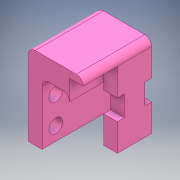
# Autodesk Inventor part: crochet
Saved by Autodesk Inventor 2017 (Build 210142000, 142)
## iProperties
Created: 2017-04-13
Part Number: crochet
Material: Generic
Document SubType Name: Modeling
Designer: franc
Density: 1 g/cm^3
Appearance: Default
Author: franc
Autodesk Inventor part; units mm, degrees
ref_plane "YZ Plane" through (0, 0, 0) normal (1, 0, 0) x (0, 1, 0)
ref_plane "XZ Plane" through (0, 0, 0) normal (0, 1, 0) x (-1, 0, 0)
ref_plane "XY Plane" through (0, 0, 0) normal (0, 0, 1) x (1, 0, 0)
sketch "Sketch1" plane through (0, 0, 0) normal (0, 1, 0) x (-1, 0, 0)
  line L0 (-4.0561, -5.7426) -> (-4.0561, 5.2574)
  line L1 (-3.0561, 6.2574) -> (2.9439, 6.2574)
  line L2 (3.9439, 5.2574) -> (3.9439, -5.7426)
  line L3 (3.9439, -5.7426) -> (1.9439, -5.7426)
  line L4 (1.9439, -5.7426) -> (1.9439, 2.2574)
  line L5 (0.9439, 3.2574) -> (-1.0561, 3.2574)
  line L6 (-2.0561, 2.2574) -> (-2.0561, -5.7426)
  line L7 (-2.0561, -5.7426) -> (-4.0561, -5.7426)
  arc A0 (-1.0561, 3.2574) -> (-2.0561, 2.2574) centre (-1.0561, 2.2574) ccw
  arc A1 (1.9439, 2.2574) -> (0.9439, 3.2574) centre (0.9439, 2.2574) ccw
  arc A2 (-3.0561, 6.2574) -> (-4.0561, 5.2574) centre (-3.0561, 5.2574) ccw
  arc A3 (3.9439, 5.2574) -> (2.9439, 6.2574) centre (2.9439, 5.2574) ccw
  point P0 (0, 0)
  point P1 (-4.0561, 6.2574)
  point P2 (3.9439, 6.2574)
  point P3 (1.9439, 3.2574)
  point P4 (-2.0561, 3.2574)
  dimension "d0" = 12
  dimension "d1" = 2
  dimension "d2" = 2
  dimension "d3" = 8
  dimension "d4" = 3
  dimension "d20" = 1
  constraints: 16 end point, 9 point on line, 8 point on circle, 8 tangent, 7 perpendicular, 4 centre point, 3 equal radius, 1 vertical
  measures "d0" distance of L0.start point (-4.056, 6.257)
  measures "d1" distance of L6.end L0.start
  measures "d2" distance of L2.end L3.end
  measures "d3" distance of point (-4.056, 6.257) point (3.944, 6.257)
  measures "d4" distance between parallel lines of L1 L5
  measures "d20" radius of A0
extrude "Extrusion1" add sketch "Sketch1" along normal blind 10
sketch "Sketch6" plane through (-1.9439, 0, 2.2574) normal (1, 0, 0) x (0, 0, -1)
  circle A0 centre (2, 2) radius 1
  circle A1 centre (6, 2) radius 1
  line L0 (8, 0) -> (8, 10) projected
  line L1 (0, 10) -> (8, 10) projected
  line L2 (8, 0) -> (0, 0) projected
  point P0 (2.2574, 0)
  dimension "d44" = 2
  dimension "d45" = 2
  dimension "d46" = 2
  dimension "d47" = 6
  dimension "d52" = 2
  dimension "d53" = 2
  constraints: 2 centre point
  measures "d44" diameter of A0
  measures "d45" diameter of A1
  measures "d46" distance from line of L0 A1.centre
  measures "d47" distance from line of L0 A0.centre
  measures "d52" distance from line of L2 A0.centre
  measures "d53" distance from line of L2 A1.centre
extrude "Extrusion6" cut sketch "Sketch6" against normal up to next
sketch "Sketch7" plane through (4.0561, 0, 5.2574) normal (1, 0, 0) x (0, 0, -1)
  line L0 (4, 10) -> (4, 9)
  line L1 (4, 9) -> (7, 9)
  line L2 (7, 9) -> (7, 10)
  line L3 (0, 10) -> (11, 10) projected
  line L4 (11, 0) -> (11, 10) projected
  line L5 (0, 0) -> (0, 10) projected
  line L6 (4, 10) -> (7, 10)
  point P0 (5.2574, 0)
  dimension "d54" = 4
  dimension "d55" = 4
  dimension "d57" = 1
  constraints: 8 end point, 2 perpendicular, 1 collinear, 1 point on line, 1 vertical
  measures "d54" distance between parallel lines of L4 L2
  measures "d55" distance between parallel lines of L5 L0
  measures "d57" distance between parallel lines of L3 L1
extrude "Extrusion7" cut sketch "Sketch7" against normal up to next
sketch "Sketch8" plane through (4.0561, 0, 5.2574) normal (1, 0, 0) x (0, 0, -1)
  line L0 (0, 0) -> (0, 10) projected
  line L1 (0, 5) -> (4, 5)
  line L2 (4, 5) -> (4, 6)
  line L3 (4, 6) -> (7, 6)
  line L4 (7, 6) -> (7, 5)
  line L5 (7, 5) -> (11, 5)
  line L6 (11, 0) -> (11, 10) projected
  line L7 (11, 5) -> (11, 0)
  line L8 (11, 0) -> (0, 0)
  line L9 (0, 0) -> (0, 5)
  point P0 (5.2574, 0)
  dimension "d60" = 5
  dimension "d61" = 1
  dimension "d62" = 4
  dimension "d63" = 4
  constraints: 16 end point, 6 perpendicular, 2 point on line, 1 horizontal, 1 midpoint
  measures "d60" distance between parallel lines of L8 L1
  measures "d61" distance of L1.end L2.end
  measures "d62" distance between parallel lines of L0 L2
  measures "d63" distance between parallel lines of L6 L4
extrude "Extrusion8" cut sketch "Sketch8" against normal up to surface (2 mm away)
body "Solid1"
